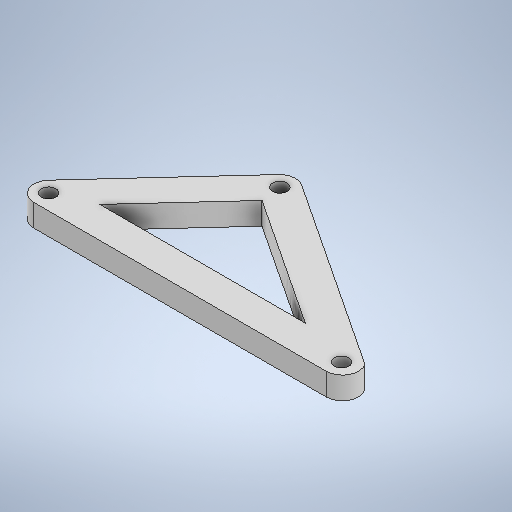
# Autodesk Inventor part: ghi
Saved by Autodesk Inventor 2025.1 (Build 291241020, 241B)
## iProperties
Created: 2025-05-24
Part Number: ghi
Material: Generic
Document SubType Name: Modeling
Designer: omiye
Density: 1 g/cm^3
Appearance: Default
Author: omiye
Autodesk Inventor part; units mm, degrees
ref_plane "YZ Plane" through (0, 0, 0) normal (1, 0, 0) x (0, 1, 0)
ref_plane "XZ Plane" through (0, 0, 0) normal (0, 1, 0) x (-1, 0, 0)
ref_plane "XY Plane" through (0, 0, 0) normal (0, 0, 1) x (1, 0, 0)
sketch "Sketch1" plane through (0, 0, 0) normal (0, 1, 0) x (-1, 0, 0)
  line L0 (0, 21.535) -> (65.7, 21.535)
  line L1 (0, 21.535) -> (40.8722, -5.4921)
  line L2 (0, 21.535) -> (49, 21.535) construction
  line L3 (40.8722, -5.4921) -> (65.7, 21.535)
  line L4 (65.7, 21.535) -> (68.7, 21.535)
  line L5 (68.7, 21.535) -> (0, 21.535)
  line L6 (0, 21.535) -> (-3, 21.535)
  line L7 (40.8722, -5.4921) -> (43.3746, -7.1468)
  line L8 (65.7, 21.535) -> (38.8426, -7.7015)
  line L9 (137.4, 18.035) -> (137.4, 25.035)
  line L10 (137.4, 25.035) -> (0, 25.035)
  line L11 (0, 25.035) -> (0, 18.035)
  line L12 (0, 18.035) -> (137.4, 18.035)
  line L13 (137.4, 18.035) -> (0, 25.035) construction
  line L14 (137.4, 25.035) -> (0, 18.035) construction
  line L15 (93.1053, 46.1943) -> (87.9503, 50.9298)
  line L16 (87.9503, 50.9298) -> (38.2947, -3.1243)
  line L17 (38.2947, -3.1243) -> (43.4497, -7.8599)
  line L18 (43.4497, -7.8599) -> (93.1053, 46.1943)
  line L19 (93.1053, 46.1943) -> (38.2947, -3.1243) construction
  line L20 (87.9503, 50.9298) -> (43.4497, -7.8599) construction
  line L21 (79.8139, -35.4386) -> (83.6749, -29.5997)
  line L22 (83.6749, -29.5997) -> (1.9305, 24.4544)
  line L23 (1.9305, 24.4544) -> (-1.9305, 18.6155)
  line L24 (-1.9305, 18.6155) -> (79.8139, -35.4386)
  line L25 (79.8139, -35.4386) -> (1.9305, 24.4544) construction
  line L26 (83.6749, -29.5997) -> (-1.9305, 18.6155) construction
  line L27 (38.8426, -7.7015) -> (38.4743, -8.1025)
  line L28 (68.7, 21.535) -> (68.7, 25.035)
  line L29 (68.7, 21.535) -> (68.7, 18.035)
  line L30 (0, 25.035) -> (-3, 25.035)
  line L31 (-3, 25.035) -> (-3, 18.035)
  line L32 (-3, 18.035) -> (0, 18.035)
  line L33 (50.67, 0) -> (41.4309, -10.0576)
  circle A0 centre (65.7, 21.535) radius 1.65
  circle A1 centre (40.8722, -5.4921) radius 1.65
  circle A2 centre (0, 21.535) radius 1.65
  point P0 (0, 0)
  point P1 (40.3135, -0.9267)
  point P2 (11.6384, 18.035)
  point P3 (57.7322, 18.035)
  point P4 (-1.0525, 18.035)
  point P5 (73.6678, 25.035)
  dimension "d0" = 65.7
  dimension "d2" = 33.475
  dimension "d3" = 3
  dimension "d4" = 3
  dimension "d7" = 39.7
  dimension "d8" = 7
  dimension "d9" = 7
  dimension "d10" = 7
  dimension "d11" = 3.3
  dimension "d12" = 3.3
  dimension "d13" = 3.3
  constraints: 68 end point, 8 midpoint, 8 point on line, 7 perpendicular, 6 parallel, 3 centre point, 3 coincident, 3 horizontal, 1 collinear, 1 equal length
  measures "d0" distance of L0.start L0.end
  measures "d2" angle of L1 L2
  measures "d3" distance of L0.end L4.end
  measures "d4" distance of L0.start L6.end
  measures "d7" distance of L0.end L8.end
  measures "d8" distance of L9.start L9.end
  measures "d9" distance of L15.start L15.end
  measures "d10" distance of L21.start L21.end
  measures "d11" diameter of A0
  measures "d12" diameter of A1
  measures "d13" diameter of A2
extrude "Extrusion1" add sketch "Sketch1" along normal blind 5 contours A2 L23 L22 L0 | L0 L22 L12 L1 A2 | L1 L12 L11 A2 | A2 L23 L24 L32 L31 L6 | L6 L31 L30 L11 A2 | L11 L10 L16 L0 L22 L23 A2 | L11 L32 L24 L23 A2 | L0 L16 L12 L22 | L12 L22 L16 L17 A1 L1 | L1 A1 L8 L27 L24 L32 L12 | L16 L10 L28 L4 A0 L0 | L0 A0 L3 L12 L16 | L12 L3 L22 L16 | L22 L3 A1 L17 L16 | A1 L17 L33 L24 L27 L8 | L10 L18 L29 L28 | L4 L29 L18 L12 L3 A0 | L12 L18 L22 L3 | L22 L18 L17 A1 L3
sketch "Sketch2" plane through (0, 5, 0) normal (0, 1, 0) x (1, 0, 0)
  line L0 (1.0525, -18.035) -> (-41.4309, 10.0576) projected
  line L1 (-41.4309, 10.0576) -> (11.6284, -25.035)
  line L2 (-41.4309, 10.0576) -> (22.1833, 10.0576) construction
  line L3 (-73.6678, -25.035) -> (3, -25.035) projected
  line L4 (11.6284, -25.035) -> (3, -25.035)
  line L5 (3, -25.035) -> (3, -18.035) projected
  line L6 (3, -18.035) -> (3, -25.035)
  point P0 (0, 0)
  point P1 (3, -19.3283)
  dimension "d16" = 33.48
  constraints: 8 end point, 2 collinear, 1 equal length, 1 horizontal
  measures "d16" angle of L1 L2
extrude "Extrusion2" add sketch "Sketch2" against normal up to surface (5 mm away)
sketch "Sketch3" plane through (0, 5, 0) normal (0, 1, 0) x (1, 0, 0)
  line L0 (3, -18.035) -> (1.0525, -18.035) projected
  line L1 (11.6284, -25.035) -> (3, -19.3283) projected
  line L2 (1.0525, -18.035) -> (3, -19.3283)
  line L3 (3, -19.3283) -> (3, -18.035)
  line L4 (3, -18.035) -> (1.0525, -18.035)
  point P0 (0, 0)
  constraints: 6 end point, 1 perpendicular, 1 vertical
extrude "Extrusion3" cut sketch "Sketch3" against normal blind 10
fillet "Fillet1" radius 3.5875 2 edges at (-73.6678, 2.5, 25.035) (-41.4309, 2.5, -10.0576)
fillet "Fillet2" radius 3.5875 1 edges at (11.6284, 2.5, 25.035)
body "Solid1"
